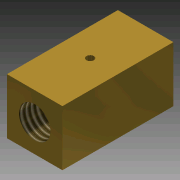
# Autodesk Inventor part: Air Release Base 1764
Saved by Autodesk Inventor 2011 (Build 150239000, 239)
## iProperties
Created: 2010-02-22
Part Number: Air Release Base 1764
Document SubType Name: Modeling
Designer: jgehrig
Density: 1 g/cm^3
Author: jgehrig
Autodesk Inventor part; units mm, degrees
ref_plane "YZ Plane" through (0, 0, 0) normal (1, 0, 0) x (0, 1, 0)
ref_plane "XZ Plane" through (0, 0, 0) normal (0, 1, 0) x (-1, 0, 0)
ref_plane "XY Plane" through (0, 0, 0) normal (0, 0, 1) x (1, 0, 0)
sketch "Sketch1" plane through (0, 0, 0) normal (0, 0, 1) x (1, 0, 0)
  line L0 (-32.8685, 12) -> (-13.8185, 12)
  line L1 (-13.8185, 12) -> (-13.8185, -7.05)
  line L2 (-13.8185, -7.05) -> (-32.8685, -7.05)
  line L3 (-32.8685, -7.05) -> (-32.8685, 12)
  circle A0 centre (-23.3435, 2.475) radius 5.3975
  point P0 (0, 0)
  dimension "d0" = 19.05
  dimension "d1" = 19.05
  dimension "d2" = 10.795
  constraints: 8 end point, 2 parallel, 1 centre point, 1 horizontal, 1 perpendicular
  measures "d0" distance of L0.start L0.end
  measures "d1" distance of L0.end L1.end
  measures "d2" diameter of A0
extrude "Extrusion1" add sketch "Sketch1" along normal blind 38.1
sketch "Sketch2" plane through (-32.8685, 12, 0) normal (0, 1, 0) x (1, 0, 0)
  circle A0 centre (9.525, -19.05) radius 1.27
  point P0 (32.8685, 0)
  dimension "d5" = 2.54
  constraints: 1 centre point
  measures "d5" diameter of A0
extrude "Extrusion2" cut sketch "Sketch2" against normal blind 6.35
thread "Thread1" size "7/16-14 UNC" class "2B" standard "ANSI Unified Screw Threads" full length
body "Solid1"
